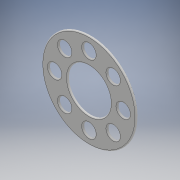
# Autodesk Inventor part: segment_1_horn_spacer
Saved by Autodesk Inventor 2018 (Build 220112000, 112)
## iProperties
Created: 2018-05-11
Part Number: segment_1_horn_spacer
Material: Generic
Document SubType Name: Modeling
Designer: mshaw2
Density: 1 g/cm^3
Appearance: Default
Author: mshaw2
## iProperties of the stored document segment_1_horn_spacer_3DPrint.ipt
Created: 2018-05-11
Part Number: segment_1_horn_spacer_3DPrint
Material: Generic
Document SubType Name: Modeling
Designer: mshaw2
Density: 1 g/cm^3
Appearance: Default
Author: mshaw2
Autodesk Inventor part; units mm, degrees
ref_plane "YZ Plane" through (0, 0, 0) normal (1, 0, 0) x (0, 1, 0)
ref_plane "XZ Plane" through (0, 0, 0) normal (0, 1, 0) x (-1, 0, 0)
ref_plane "XY Plane" through (0, 0, 0) normal (0, 0, 1) x (1, 0, 0)
sketch "Sketch1" plane through (0, 0, 0) normal (0, 1, 0) x (-1, 0, 0)
  circle A0 centre (-5.6569, 5.6569) radius 1.45
  circle A1 centre (0, 8) radius 1.45
  circle A2 centre (5.6569, 5.6569) radius 1.45
  circle A3 centre (8, 0) radius 1.45
  circle A4 centre (5.6569, -5.6569) radius 1.45
  circle A5 centre (0, -8) radius 1.45
  circle A6 centre (-5.6569, -5.6569) radius 1.45
  circle A7 centre (-8, 0) radius 1.45
  circle A8 centre (0, 0) radius 5
  circle A9 centre (0, 0) radius 11
  constraints: 10 centre point
extrude "Extrusion1" add sketch "Sketch1" along normal blind 0.5
fillet "Fillet1" radius 0.25 20 edges at (1.45, 0.5, 8) (1.45, 0, 8) (5, 0, 0) (5, 0.5, 0) (11, 0.5, 0) (11, 0, 0) (7.1069, 0.5, -5.6569) (7.1069, 0, -5.6569) (9.45, 0, 0) (9.45, 0.5, 0) (7.1069, 0.5, 5.6569) (7.1069, 0, 5.6569) (-6.55, 0, 0) (-6.55, 0.5, 0) (-4.2069, 0, 5.6569) (-4.2069, 0.5, 5.6569) (-4.2069, 0.5, -5.6569) (-4.2069, 0, -5.6569) (1.45, 0.5, -8) (1.45, 0, -8)
body "Solid1"
